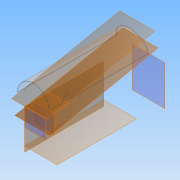
# Autodesk Inventor part: Top_Guard 1
Saved by Autodesk Inventor 2018.1 (Build 221171000, 171)
## iProperties
Created: 2019-03-23
Part Number: Top_Guard 1
Material: PMMA Plastic
Document SubType Name: Modeling
Designer: James
Density: 1.188 g/cm^3
Appearance: Polycarbonate - Clear
Author: James
Autodesk Inventor part; units mm, degrees
ref_plane "YZ Plane" through (0, 0, 0) normal (1, 0, 0) x (0, 1, 0)
ref_plane "XZ Plane" through (0, 0, 0) normal (0, 1, 0) x (-1, 0, 0)
ref_plane "XY Plane" through (0, 0, 0) normal (0, 0, 1) x (1, 0, 0)
derived "Top_Skeleton.ipt"
ref_plane "Work Plane1" through (0, 0, 0) normal (0, 0, 1) x (1, 0, 0)
ref_plane "Work Plane2" through (0, 0, 0) normal (0, 1, 0) x (-1, 0, 0)
ref_plane "Work Plane3" through (0, 0, 0) normal (1, 0, 0) x (0, 1, 0)
ref_plane "Work Plane4" through (0, 4100, 0) normal (0, 1, 0) x (-1, 0, 0)
ref_plane "Work Plane5" through (0, 0, -1300) normal (0, 0, 1) x (1, 0, 0)
ref_plane "Work Plane6" through (0, 325, 0) normal (0, 1, 0) x (-1, 0, 0)
sketch "Sketch1" plane through (0, 325, 0) normal (0, 1, 0) x (-1, 0, 0)
  arc A0 (610, 0) -> (-610, 0) centre (0, 0) ccw
  arc A1 (600, 0) -> (-600, 0) centre (0, 0) ccw
  line L0 (610, 0) -> (600, 0)
  line L1 (-600, 0) -> (-610, 0)
  dimension "d0" = 1200
  dimension "d1" = 10
  constraints: 4 end point, 4 point on circle, 2 centre point, 2 coincident, 2 horizontal alignment, 1 collinear, 1 horizontal
  measures "d0" diameter of A1
  measures "d1" radial gap between concentric circles of A0 A1
extrude "Extrusion1" add sketch "Sketch1" along normal up to surface (3775 mm away)
sketch "Sketch2" plane through (0, 0, 0) normal (1, 0, 0) x (0, 1, 0)
  line L0 (4100, 610) -> (4100, 0) projected
  line L1 (325, 0) -> (4100, 0) projected
  line L2 (4100, 0) -> (4100, 600) projected
  line L3 (4100, 0) -> (3896.5477, 1000)
  line L4 (3896.5477, 1000) -> (4100, 1000)
  line L5 (4100, 1000) -> (4100, 0)
  point P0 (0, 0)
  dimension "d6" = 11.5
  dimension "d7" = 1000
  constraints: 6 end point, 1 collinear, 1 perpendicular
  measures "d6" angle of L0 L3
  measures "d7" distance from line of L0.end L4
extrude "Extrusion2" cut sketch "Sketch2" along normal through all both and the other way through all
sketch "Sketch4" plane through (0, 0, 0) normal (1, 0, 0) x (0, 1, 0)
  circle A0 centre (970, 0) radius 150
  line L0 (325, 0) -> (325, 610) projected
  line L1 (325, 0) -> (4100, 0) projected
  line L2 (0, 762) -> (0, -302) projected
  point P0 (0, 0)
  dimension "d12" = 300
  dimension "d16" = 970
  constraints: 1 centre point, 1 point on line
  measures "d12" diameter of A0
  measures "d16" distance from line of A0.centre L2
extrude "Extrusion3" cut sketch "Sketch4" along normal through all
sketch "Sketch6" plane through (0, 0, 0) normal (0, 0, 1) x (1, 0, 0)
  line L0 (610, 325) -> (-610, 325) projected
  line L1 (0, 4920) -> (0, -820) projected
  point P0 (0, 0)
  point P1 (0, 330)
  dimension "d17" = 5
  constraints: 1 point on line
  measures "d17" distance from line of L0 point (0, 330)
hole "Hole1" at (0, 330, 0) direction (0, 0, 1) diameter 4.5 end through all clearance for "Flat Head Machine Screw" size "M4" standard "Ansi Metric M Profile"
pattern_circular "Circular Pattern1" count 14 over 360 about axis through (0, -10, 0) along (0, 1, 0) of "Hole1"
ref_plane "Work Plane7" through (305, 4100, 0) normal (0, -0.1993679, 0.9799247) x (1, 0, 0)
ref_plane "Work Plane8" through (305, 3974.3982, 617.3526) normal (0, -0.1993679, 0.9799247) x (1, 0, 0)
sketch "Sketch7" plane through (305, 3974.3982, 617.3526) normal (0, -0.1993679, 0.9799247) x (1, 0, 0)
  line L0 (-915, 0) -> (305, 0) projected
  line L1 (-305, 951.2346) -> (-305, -4845.8456) projected
  point P0 (-305, -4017.6913)
  point P1 (-305, -5)
  dimension "d30" = 5
  constraints: 1 point on line
  measures "d30" distance from line of point (-305, -5) L0
hole "Hole2" at (0, 3969.4986, 616.3557) direction (0, 0.1993679, -0.9799247) diameter 4.5 depth 50 tip angle 118 clearance for "Flat Head Machine Screw" size "M4" standard "Ansi Metric M Profile"
ref_plane "Work Plane9" through (305, 4099.6013, 1.9598) normal (0, -0.1993679, 0.9799247) x (1, 0, 0)
pattern_circular "Circular Pattern2" count 14 over 360 about axis through (0, 4099.6013, 1.9598) along (0, 0.9799247, 0.1993679) of "Hole2"
body "Solid1"
